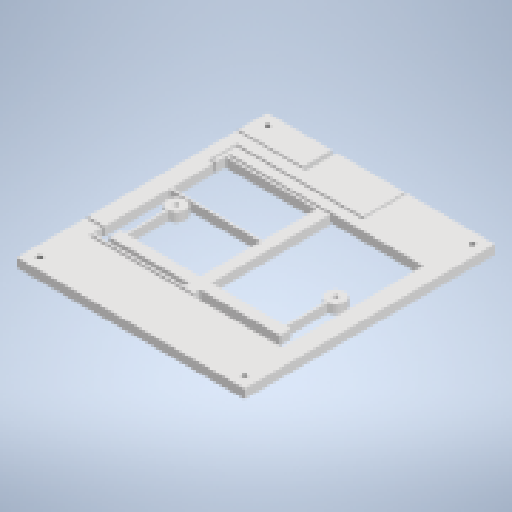
# Autodesk Inventor part: FlexK7Holder
Saved by Autodesk Inventor 2023 (Build 270158000, 158)
## iProperties
Created: 2023-03-30
Part Number: FlexK7Holder
Material: Generic
Document SubType Name: Modeling
Designer: Nathann
Density: 1 g/cm^3
Appearance: Default
Author: Nathann
Autodesk Inventor part; units mm, degrees
ref_plane "YZ Plane" through (0, 0, 0) normal (1, 0, 0) x (0, 1, 0)
ref_plane "XZ Plane" through (0, 0, 0) normal (0, 1, 0) x (-1, 0, 0)
ref_plane "XY Plane" through (0, 0, 0) normal (0, 0, 1) x (1, 0, 0)
sketch "Sketch1" plane through (0, 0, 0) normal (0, 1, 0) x (-1, 0, 0)
  line L0 (0, 0) -> (-100, 0)
  line L1 (-100, 0) -> (-100, -110)
  line L2 (-100, -110) -> (0, -110)
  line L3 (0, -110) -> (0, 0)
  dimension "d0" = 110
  dimension "d1" = 100
  constraints: 8 end point, 2 parallel, 1 horizontal, 1 perpendicular
  measures "d0" distance of L0.end L1.end
  measures "d1" distance of L0.start L0.end
extrude "Extrusion1" add sketch "Sketch1" along normal blind 4
sketch "Sketch5" plane through (0, 4, 0) normal (0, 1, 0) x (1, 0, 0)
  circle A0 centre (5, 5) radius 1.1
  line L0 (0, 0) -> (100, 0) projected
  line L1 (0, 110) -> (0, 0) projected
  line L2 (0, 55) -> (10.2566, 55)
  circle A1 centre (5, 105) radius 1.1
  line L3 (0, 110) -> (100, 110)
  line L4 (0, 0) -> (0, 110)
  line L5 (50, 0) -> (50, 7.5266)
  circle A2 centre (95, 5) radius 1.1
  line L6 (100, 110) -> (100, 0)
  circle A3 centre (95, 105) radius 1.1
  line L7 (100, 0) -> (100, 110)
  point P0 (100, 55)
  point P1 (89.7434, 55)
  dimension "d41" = 5
  dimension "d42" = 5
  dimension "d43" = 2.2
  constraints: 12 end point, 12 symmetric about line, 4 centre point, 2 midpoint, 1 horizontal, 1 vertical, 3 other
  measures "d41" distance from line of L0 A0.centre
  measures "d42" distance from line of A0.centre L1
  measures "d43" diameter of A0
extrude "Extrusion4" cut sketch "Sketch5" against normal blind 10 contours A0 | A1 | A2 | A3
thread "Thread7" size "M2.5x0.45" class "6H" standard "ANSI Metric M Profile" length 10
thread "Thread8" size "M2.5x0.45" class "6H" standard "ANSI Metric M Profile" length 10
thread "Thread9" size "M2.5x0.45" class "6H" standard "ANSI Metric M Profile" length 10
thread "Thread10" size "M2.5x0.45" class "6H" standard "ANSI Metric M Profile" length 10
sketch "Sketch6" plane through (0, 0, 0) normal (0, -1, 0) x (1, 0, 0)
  line L0 (0, 0) -> (100, 0) projected
  line L1 (0, -110) -> (0, 0) projected
  line L2 (47.5, -85) -> (52.5, -85)
  line L3 (52.5, -85) -> (52.5, -25)
  line L4 (52.5, -25) -> (47.5, -25)
  line L5 (47.5, -25) -> (47.5, -85)
  line L6 (47.5, -85) -> (52.5, -25) construction
  line L7 (52.5, -85) -> (47.5, -25) construction
  line L8 (100, 0) -> (100, -110) projected
  line L9 (100, -110) -> (0, -110) projected
  line L10 (47.5, -25) -> (7.5, -25)
  line L11 (7.5, -25) -> (7.5, -26)
  line L12 (7.5, -26) -> (47.5, -26)
  line L13 (47.5, -26) -> (47.5, -25)
  line L14 (47.5, -85) -> (7.5, -85)
  line L15 (7.5, -85) -> (7.5, -84)
  line L16 (7.5, -84) -> (47.5, -84)
  line L17 (47.5, -84) -> (47.5, -85)
  line L18 (52.5, -33) -> (52.5, -28)
  circle A0 centre (15, -55) radius 1.1
  line L19 (7.5, -26) -> (7.5, -84)
  line L20 (92.5, -28) -> (92.5, -85)
  line L21 (92.5, -85) -> (52.5, -85)
  line L22 (52.5, -85) -> (52.5, -28)
  line L23 (7.5, -25) -> (92.5, -25)
  line L24 (92.5, -25) -> (92.5, -24)
  line L25 (92.5, -24) -> (7.5, -24)
  line L26 (7.5, -24) -> (7.5, -25)
  line L27 (7.5, -85) -> (92.5, -85)
  line L28 (92.5, -85) -> (92.5, -86)
  line L29 (92.5, -86) -> (7.5, -86)
  line L30 (7.5, -86) -> (7.5, -85)
  line L31 (92.5, -28) -> (92.5, -25)
  line L32 (47.5, -60.5) -> (7.5, -60.5)
  line L33 (7.5, -60.5) -> (7.5, -59.5)
  line L34 (7.5, -59.5) -> (47.5, -59.5)
  line L35 (47.5, -59.5) -> (47.5, -60.5)
  line L36 (47.5, -28) -> (12.5, -28)
  line L37 (12.5, -28) -> (12.5, -33)
  line L38 (12.5, -33) -> (47.5, -33)
  line L39 (47.5, -33) -> (47.5, -28)
  arc A1 (14.5, -51.0314) -> (15.5, -51.0314) centre (15, -55) ccw
  line L40 (14.5, -33) -> (15.5, -33)
  line L41 (15.5, -33) -> (15.5, -51.0314)
  line L42 (14.5, -51.0314) -> (14.5, -33)
  line L43 (50, -85) -> (50, -73.5088)
  circle A2 centre (85, -55) radius 1.1
  line L44 (52.5, -28) -> (87.5, -28)
  line L45 (87.5, -28) -> (87.5, -33)
  line L46 (87.5, -33) -> (52.5, -33)
  line L47 (52.5, -33) -> (52.5, -28)
  arc A3 (84.5, -51.0314) -> (85.5, -51.0314) centre (85, -55) ccw
  line L48 (85.5, -33) -> (84.5, -33)
  line L49 (84.5, -33) -> (84.5, -51.0314)
  line L50 (85.5, -51.0314) -> (85.5, -33)
  point P0 (50, -55)
  point P1 (47.5, -59.5)
  point P2 (15.5, -42.2901)
  point P3 (15, -51.5803)
  point P4 (84.5, -42.2901)
  point P5 (85, -51.5803)
  point P6 (52.5, -25)
  point P7 (47.5, -59.5)
  dimension "d113" = 50
  dimension "d115" = 5
  dimension "d117" = 1
  dimension "d119" = 40
  dimension "d121" = 40
  dimension "d122" = 1
  dimension "d140" = 2.2
  dimension "d141" = 40
  dimension "d142" = 1
  dimension "d143" = 1
  dimension "d151" = 1
  dimension "d166" = 35
  dimension "d167" = 55
  dimension "d168" = 35
  dimension "d169" = 5
  dimension "d170" = 2
  dimension "d171" = 8
  dimension "d172" = 1
  dimension "d173" = 0
  constraints: 94 end point, 16 parallel, 9 point on line, 8 horizontal, 8 perpendicular, 8 symmetric about line, 4 centre point, 4 point on circle, 3 midpoint, 3 vertical, 2 coincident, 2 other
  measures "d113" distance from line of L8 point (50, -55)
  measures "d115" distance of L3.end L4.end
  measures "d117" distance between parallel lines of L10 L12
  measures "d119" distance of L4.end L10.end
  measures "d121" distance of L2.start L14.end
  measures "d122" distance between parallel lines of L14 L16
  measures "d140" diameter of A0
  measures "d141" distance between parallel lines of L22 L20
  measures "d142" distance between parallel lines of L27 L29
  measures "d143" distance between parallel lines of L25 L23
  measures "d151" distance between parallel lines of L32 L34
  measures "d166" distance of point (50, -55) A0.centre
  measures "d167" distance from line of L9 A0.centre
  measures "d168" distance of L37.end L38.end
  measures "d169" distance of L36.end L37.end
  measures "d170" distance between parallel lines of L12 L36
  measures "d171" diameter of A1
  measures "d172" distance from line of point (15.5, -42.29) L42
  measures "d173" horizontal distance of A0.centre point (15, -51.58)
extrude "Extrusion5" cut sketch "Sketch6" against normal blind 4 contours L2 L21 L28 L29 L30 L14 | L16 L19 L32 L5 | L3 L46 L49 A3 L50 L45 L44 L23 L31 L20 L21 | L34 L19 L12 L5 L36 L37 L38 L42 A1 L41 | L4 L10 L26 L25 L24 L23 | A0 | A2
sketch "Sketch8" plane through (0, 4, 0) normal (0, 1, 0) x (1, 0, 0)
  line L0 (100, 110) -> (0, 110) projected
  line L1 (60.5042, 110) -> (30.5042, 110)
  line L2 (30.5042, 110) -> (30.5042, 96.3922)
  line L3 (30.5042, 96.3922) -> (60.5042, 96.3922)
  line L4 (60.5042, 96.3922) -> (60.5042, 110)
  line L5 (0, 110) -> (0, 0) projected
  line L6 (60.5042, 96.3922) -> (0, 96.3922)
  line L7 (0, 96.3922) -> (0, 91.3922)
  line L8 (0, 91.3922) -> (60.5042, 91.3922)
  line L9 (60.5042, 91.3922) -> (60.5042, 96.3922)
  line L10 (0, 91.3922) -> (5, 91.3922)
  line L11 (5, 91.3922) -> (5, 31)
  line L12 (5, 31) -> (0, 31)
  line L13 (0, 31) -> (0, 91.3922)
  line L14 (7.5, 60.5) -> (7.5, 84) projected
  line L15 (5, 31) -> (7.5, 31)
  line L16 (7.5, 31) -> (7.5, 79)
  line L17 (7.5, 79) -> (5, 79)
  line L18 (5, 79) -> (5, 31)
  line L19 (7.5, 84) -> (47.5, 84) projected
  line L20 (47.5, 26) -> (7.5, 26) projected
  line L21 (7.5, 80) -> (6, 80)
  line L22 (6, 80) -> (6, 90.3922)
  line L23 (6, 90.3922) -> (61.5042, 90.3922)
  line L24 (61.5042, 90.3922) -> (61.5042, 110)
  line L25 (0, 97.2327) -> (28.374, 97.2327)
  line L26 (28.374, 97.2327) -> (28.374, 110)
  line L27 (7.5, 26) -> (7.5, 59.5) projected
  line L28 (7.5, 30) -> (0, 30)
  point P0 (6.25, 79)
  point P1 (0, 31)
  point P2 (0, 96.3922)
  point P3 (5, 91.3922)
  dimension "d153" = 5
  dimension "d154" = 5
  dimension "d155" = 5
  dimension "d156" = 5
  dimension "d157" = 30
  dimension "d158" = 1
  dimension "d159" = 1
  dimension "d160" = 1
  dimension "d161" = 1
  dimension "d162" = 1
  constraints: 46 end point, 9 parallel, 9 point on line, 8 perpendicular, 6 horizontal, 1 midpoint
  measures "d153" distance between parallel lines of L19 L17
  measures "d154" distance between parallel lines of L15 L20
  measures "d155" distance between parallel lines of L5 L11
  measures "d156" distance between parallel lines of L8 L6
  measures "d157" distance between parallel lines of L2 L4
  measures "d158" distance from line of L28 L11.end
  measures "d159" distance from line of point (6.25, 79) L21
  measures "d160" distance between parallel lines of L11 L22
  measures "d161" distance between parallel lines of L23 L8
  measures "d162" distance between parallel lines of L24 L4
extrude "Extrusion6" cut sketch "Sketch8" against normal blind 4 contours L24 L23 L22 L21 L14 L17 L11 L8 L9 L4 L0 | L2 L6 L5 L25 L26 L0 | L12 L15 L27 L28 L5
body "Solid1"
